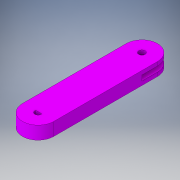
# Autodesk Inventor part: Arm
Saved by Autodesk Inventor 2017 (Build 210142000, 142)
## iProperties
Created: 2017-03-25
Part Number: Arm
Material: Generic
Document SubType Name: Modeling
Designer: Parshant Bombhi
Density: 1 g/cm^3
Appearance: Default
LengthOfArm_Thiner: 6.500 in
Thickness_Thiner: 0.625 in
Author: Parshant Bombhi
Autodesk Inventor part; units mm, degrees
ref_plane "YZ Plane" through (0, 0, 0) normal (1, 0, 0) x (0, 1, 0)
ref_plane "XZ Plane" through (0, 0, 0) normal (0, 1, 0) x (-1, 0, 0)
ref_plane "XY Plane" through (0, 0, 0) normal (0, 0, 1) x (1, 0, 0)
sketch "Sketch1" plane through (0, 0, 0) normal (0, 1, 0) x (-1, 0, 0)
  line L0 (0, -19.05) -> (0, -146.05)
  line L1 (19.05, -165.1) -> (19.05, -165.1)
  line L2 (38.1, -146.05) -> (38.1, -19.05)
  line L3 (19.05, 0) -> (19.05, 0)
  arc A0 (0, -146.05) -> (19.05, -165.1) centre (19.05, -146.05) ccw
  arc A1 (19.05, -165.1) -> (38.1, -146.05) centre (19.05, -146.05) ccw
  arc A2 (38.1, -19.05) -> (19.05, 0) centre (19.05, -19.05) ccw
  arc A3 (19.05, 0) -> (0, -19.05) centre (19.05, -19.05) ccw
  circle A4 centre (19.05, -19.05) radius 3.9688
  circle A5 centre (19.05, -146.05) radius 3.9688
  point P0 (0, 0)
  point P1 (0, -165.1)
  point P2 (38.1, -165.1)
  dimension "d0" = 38.1
  dimension "LengthOfArm_Thiner" = 165.1
  dimension "d2" = 19.05
  dimension "Motor_Shaft_Diameter" = 7.9375
  dimension "d4" = 7.9375
  constraints: 8 end point, 8 point on circle, 8 tangent, 6 centre point, 6 point on line, 3 equal radius, 3 perpendicular, 2 coincident, 1 vertical
  measures "d0" distance of point (0, -165.1) point (38.1, -165.1)
  measures "LengthOfArm_Thiner" distance of point (0, 0) point (0, -165.1)
  measures "d2" radius of A0
  measures "Motor_Shaft_Diameter" diameter of A4
  measures "d4" diameter of A5
extrude "Extrusion1" add sketch "Sketch1" along normal blind 15.875
sketch "Sketch2" plane through (-38.1, 0, -146.05) normal (-1, 0, 0) x (0, 0, 1)
  line L0 (-19.05, 0) -> (-19.05, 15.875) projected
  line L1 (-57.15, 4.7625) -> (19.05, 4.7625)
  line L2 (19.05, 4.7625) -> (19.05, 11.1125)
  line L3 (19.05, 11.1125) -> (-57.15, 11.1125)
  line L4 (-57.15, 11.1125) -> (-57.15, 4.7625)
  line L5 (-57.15, 4.7625) -> (19.05, 11.1125) construction
  line L6 (19.05, 4.7625) -> (-57.15, 11.1125) construction
  point P0 (146.05, 0)
  point P1 (-19.05, 7.9375)
  dimension "d7" = 6.35
  dimension "d8" = 38.1
  constraints: 12 end point, 3 midpoint, 2 parallel, 1 horizontal, 1 perpendicular
  measures "d7" distance of L1.end L2.end
  measures "d8" distance from line of L2 point (-19.05, 7.938)
extrude "Extrusion2" cut sketch "Sketch2" against normal up to next
sketch "Sketch3" plane through (0, 15.875, 0) normal (0, 1, 0) x (1, 0, 0)
  circle A0 centre (-19.05, 19.05) radius 3.9687 projected
  line L0 (-24.4521, 26.1937) -> (-13.6479, 26.1937)
  line L1 (-13.6479, 26.1937) -> (-13.6479, 19.8437)
  line L2 (-13.6479, 19.8437) -> (-24.4521, 19.8437)
  line L3 (-24.4521, 19.8437) -> (-24.4521, 26.1937)
  line L4 (-24.4521, 26.1937) -> (-13.6479, 19.8437) construction
  line L5 (-13.6479, 26.1937) -> (-24.4521, 19.8437) construction
  point P0 (0, 0)
  point P1 (-19.05, 23.0187)
  dimension "d11" = 6.35
  constraints: 12 end point, 2 midpoint, 2 parallel, 1 coincident, 1 horizontal, 1 perpendicular, 1 vertical alignment, 1 other
  measures "d11" distance of L0.end L1.end
extrude "Extrusion3" add sketch "Sketch3" against normal up to surface (15.875 mm away) contours L2 A0 | A0 L2 L3 L0 L1 picked at (-18.8857, 21.5143)
body "Solid1"
